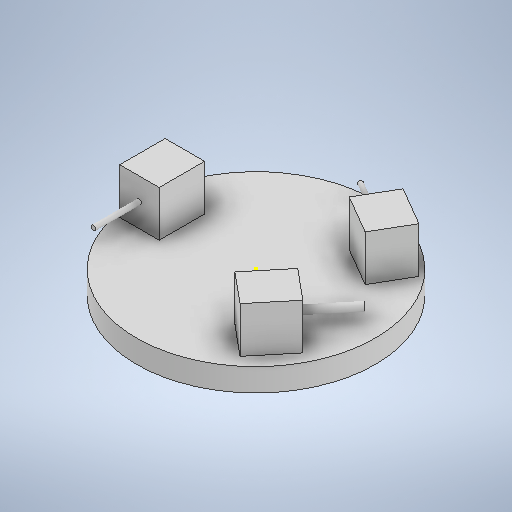
# Autodesk Inventor part: Base
Saved by Autodesk Inventor 2025 (Build 290162000, 162)
## iProperties
Created: 2025-04-15
Part Number: Base
Material: Generic
Document SubType Name: Modeling
Designer: hp
Density: 1 g/cm^3
Appearance: Default
Author: hp
Autodesk Inventor part; units mm, degrees
ref_plane "YZ Plane" through (0, 0, 0) normal (1, 0, 0) x (0, 1, 0)
ref_plane "XZ Plane" through (0, 0, 0) normal (0, 1, 0) x (-1, 0, 0)
ref_plane "XY Plane" through (0, 0, 0) normal (0, 0, 1) x (1, 0, 0)
sketch "Sketch1" plane through (0, 0, 0) normal (0, 1, 0) x (-1, 0, 0)
  circle A0 centre (0, 0) radius 13.2908
  line L0 (0, 0) -> (-6.6454, 11.5102)
  line L1 (0, 0) -> (13.2908, 0) construction
  line L2 (0, 0) -> (-6.6454, -11.5102)
  constraints: 6 end point, 2 point on circle, 1 centre point, 1 coincident, 1 equal length, 1 horizontal
extrude "Extrusion1" add sketch "Sketch1" against normal blind 2.54
sketch "Sketch2" plane through (0, 0, 0) normal (0, 1, 0) x (1, 0, 0)
  line L0 (-12.5731, -2.5944) -> (-8.1825, -2.5944)
  line L1 (-8.1825, -2.5944) -> (-8.1825, 2.4614)
  line L2 (-8.1825, 2.4614) -> (-12.5731, 2.4614)
  line L3 (-12.5731, 2.4614) -> (-12.5731, -2.5944)
  line L4 (4.1689, -6.5202) -> (7.5172, -9.2912)
  line L5 (7.5172, -9.2912) -> (10.6841, -5.4645)
  line L6 (10.6841, -5.4645) -> (7.3357, -2.6935)
  line L7 (7.3357, -2.6935) -> (4.1689, -6.5202)
  line L8 (5.5175, 10.8555) -> (3.3095, 7.0709)
  line L9 (3.3095, 7.0709) -> (7.5616, 4.5902)
  line L10 (7.5616, 4.5902) -> (9.7696, 8.3747)
  line L11 (9.7696, 8.3747) -> (5.5175, 10.8555)
  point P0 (0, 0)
  constraints: 24 end point, 6 parallel, 3 perpendicular, 1 horizontal
extrude "Extrusion2" add sketch "Sketch2" along normal blind 5.08
sketch "Sketch3" plane through (7.3357, 0, 2.6935) normal (0.6376, 0, -0.7704) x (-0.7704, 0, -0.6376)
  circle A0 centre (-2.0466, 2.54) radius 0.4266
  point P0 (7.3687, 0)
  constraints: 1 centre point
extrude "Extrusion3" add sketch "Sketch3" along normal blind 5.08
sketch "Sketch4" plane through (3.3095, 0, -7.0709) normal (-0.8637, 0, -0.5039) x (-0.5039, 0, 0.8637)
  circle A0 centre (-2.246, 2.54) radius 0.2524
  point P0 (7.7752, 0)
  constraints: 1 centre point
extrude "Extrusion4" add sketch "Sketch4" along normal blind 5.08
sketch "Sketch5" plane through (-12.5731, 0, 2.5944) normal (0, 0, 1) x (1, 0, 0)
  circle A0 centre (2.148, 2.6) radius 0.2719
  point P0 (12.5731, 0)
  constraints: 1 centre point
extrude "Extrusion5" add sketch "Sketch5" along normal blind 5.08
sketch "Sketch6" plane through (0, 0, 0) normal (0, 1, 0) x (1, 0, 0)
  point P0 (0, 0)
body "Solid1"
